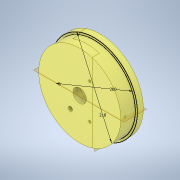
# Autodesk Inventor part: insulation_lid_objective
Saved by Autodesk Inventor 2020.2 (Build 242310000, 310)
## iProperties
Created: 2019-03-06
Part Number: insulation_lid_objective
Material: ABS Plastic light yellow
Document SubType Name: Modeling
Designer: rainer
Density: 1.06 g/cm^3
Appearance: Smooth - White
Mass: 1012.79 g
Surface Area: 1136.06 cm^2
Volume: 955.458 cm^3
Author: rainer
Autodesk Inventor part; units mm, degrees
ref_plane "XZ Plane" through (0, 0, 0) normal (0, 1, 0) x (-1, 0, 0)
ref_plane "XY Plane" through (0, 0, 0) normal (0, 0, 1) x (1, 0, 0)
sketch "Sketch1" plane through (0, 0, 0) normal (0, 0, 1) x (1, 0, 0)
  circle A0 centre (0, 0) radius 100
  circle A1 centre (0, 0) radius 105
  dimension "d0" = 200
  dimension "d48" = 210
  constraints: 2 centre point, 2 coincident
  measures "d0" diameter of A0
  measures "d48" diameter of A1
extrude "Extrusion1" add sketch "Sketch1" along normal blind 35 contours A0
sketch "Sketch2" plane through (0, 0, 0) normal (0, 0, -1) x (-1, 0, 0)
  circle A0 centre (0, 0) radius 90.5
  circle A1 centre (0, 0) radius 60
  dimension "d3" = 181
  dimension "d4" = 120
  constraints: 2 centre point, 2 coincident
  measures "d3" diameter of A0
  measures "d4" diameter of A1
extrude "Extrusion2" cut sketch "Sketch2" against normal blind 10
sketch "Sketch3" plane through (0, 0, 0) normal (0, 0, -1) x (-1, 0, 0)
  circle A0 centre (-50, 0) radius 2.5
  line L0 (0, 0) -> (22.5, -38.9711)
  line L1 (0, 0) -> (45, 0) construction
  line L2 (0, 0) -> (-50, 0)
  dimension "d7" = 5
  dimension "d8" = 50
  dimension "d23" = 45
  dimension "d24" = 60
  constraints: 6 end point, 1 centre point, 1 collinear, 1 equal length, 1 horizontal
  measures "d7" diameter of A0
  measures "d8" distance of L0.start L2.end
  measures "d23" distance of L0.start L0.end
  measures "d24" angle of L0 L1
extrude "Extrusion3" cut sketch "Sketch3" against normal blind 25
ref_plane "Work Plane1" through (100, 0, 0) normal (1, 0, 0) x (0, 1, 0)
sketch "Sketch4" plane through (100, 0, 0) normal (1, 0, 0) x (0, 1, 0)
  circle A0 centre (0, 25) radius 2.5
  line L0 (-100, 0) -> (100, 0) projected
  point P0 (0, 0)
  dimension "d12" = 5
  dimension "d13" = 25
  constraints: 1 centre point
  measures "d12" diameter of A0
  measures "d13" distance from line of L0 A0.centre
extrude "Extrusion4" cut sketch "Sketch4" against normal blind 52.5
sketch "Sketch5" plane through (0, 0, 35) normal (0, 0, 1) x (1, 0, 0)
  circle A0 centre (0, 0) radius 16.25
  dimension "d16" = 32.5
  constraints: 1 centre point, 1 coincident
  measures "d16" diameter of A0
extrude "Extrusion5" cut sketch "Sketch5" against normal blind 50
thicken "Thicken1" operation add thickness 15 both sides no extend neighbours yes toward (0, 0, -1) faces at (-1.2192, -96.6103, 0)
thicken "Thicken2" operation add thickness 5 both sides no extend neighbours yes toward (0, 0, 1) faces at (38.8585, -11.7475, 0)
hole "Hole1" at (-22.5, -38.9711, 0) direction (0, 0, 1) diameter 10 end through all
extrude "Extrusion7" add sketch "Sketch1" against normal up to surface (15 mm away)
ref_plane "Work Plane2" through (0, 0, 0) normal (0, 1, 0) x (1, 0, 0)
sketch "Sketch7" plane through (0, 0, 0) normal (0, 1, 0) x (1, 0, 0)
  line L0 (-100, -35) -> (100, -35) projected
  line L1 (0, -35) -> (30, -35)
  line L2 (30, -35) -> (30, -17)
  line L3 (30, -17) -> (-35, -17)
  line L4 (-35, -17) -> (-35, 15)
  line L5 (100, 15) -> (-100, 15) projected
  dimension "d36" = 30
  dimension "d37" = 18
  dimension "d38" = 65
  constraints: 8 end point, 3 perpendicular, 2 point on line, 1 midpoint
  measures "d36" distance of L1.start L1.end
  measures "d37" distance of L1.end L2.end
  measures "d38" distance of L2.end L3.end
ref_plane "Work Plane3" through (30, -95.3939, 17) normal (-1, 0, 0) x (0, 0, 1)
split body "Split6" sketch "Sketch7" result two bodies curves L1 L2 L3 L4 first body at (-47.5044, -14.9713, 34.5)
sketch "Sketch9" plane through (0, 0, 35) normal (0, 0, 1) x (1, 0, 0)
  line L0 (18.1747, 51.3397) -> (-55.7483, 8.6603)
  arc A0 (-55.7483, 8.6603) -> (-55.7483, -8.6603) centre (-50.7483, 0) ccw
  line L1 (-55.7483, -8.6603) -> (18.1747, -51.3397)
  arc A1 (18.1747, -51.3397) -> (33.1747, -36.0471) centre (24.641, -42.6795) ccw
  line L2 (33.1747, -36.0471) -> (33.1747, 49.3119)
  arc A2 (33.1747, 49.3119) -> (18.1747, 51.3397) centre (24.641, 42.6795) ccw
  line L3 (24.641, 42.6795) -> (24.641, -42.6795) construction
  circle A3 centre (-50.7483, 0) radius 1.5 construction
  line L4 (-50.7483, 0) -> (24.641, 0) construction
  line L5 (24.641, 42.6795) -> (-49.282, 0) construction
  line L6 (24.641, -42.6795) -> (-12.3205, 21.3397) construction
  line L7 (-49.282, 0) -> (24.641, -42.6795) construction
  line L8 (24.641, 42.6795) -> (-12.3205, -21.3397) construction
  circle A4 centre (0, 0) radius 17.5
  dimension "d53" = 35
  dimension "d61" = 0
  dimension "d62" = 0
  constraints: 18 end point, 6 point on circle, 5 centre point, 3 midpoint, 3 point on line, 1 coincident, 1 vertical
  measures "d53" diameter of A4
  measures "d61" distance of point (0, 0) A4.centre
  measures "d62" distance of point (0, 0) A4.centre
hole "Hole2" at (-49.282, 0, 35) at (24.641, -42.6795, 35) at (24.641, 42.6795, 35) direction (0, 0, -1) diameter 6 depth 30 bodies 2 3
sketch "Sketch8" plane through (30, -95.3939, 17) normal (-1, 0, 0) x (0, 0, 1)
  line L0 (18, 95.3939) -> (18, 190.7878) projected
  line L1 (18, 95.3939) -> (18, 125.3939)
  line L2 (18, 125.3939) -> (9, 125.3939)
  line L3 (9, 125.3939) -> (9, 65.3939)
  circle A0 centre (9, 125.3939) radius 4
  circle A1 centre (9, 65.3939) radius 4
  point P0 (-17, 95.3939)
  dimension "d39" = 30
  dimension "d40" = 9
  dimension "d41" = 60
  dimension "d42" = 8
  dimension "d43" = 8
  constraints: 6 end point, 2 centre point, 2 coincident, 2 perpendicular, 1 point on line
  measures "d39" distance of L0.start L1.end
  measures "d40" distance of L1.end L2.end
  measures "d41" distance of L2.end L3.end
  measures "d42" diameter of A0
  measures "d43" diameter of A1
extrude "Extrusion8" cut sketch "Sketch8" along normal mid plane 40 bodies 2 3
body "Solid8"
body "Solid9"
